Autodesk Fusion 360 part; units mm, degrees
(part 2 of 2)
sketch "草图2" plane through (0, 0, 0) normal (0, 0, 1) x (1, 0, 0)
  circle A0 centre (-78, 71) radius 2.1
  circle A1 centre (0, 135) radius 5
  circle A2 centre (-78, 101) radius 2.1
  circle A3 centre (6, 76.5) radius 1.5
  circle A4 centre (53, 101) radius 2.1
  arc A5 (8, 81) -> (8, 91) centre (8, 86) ccw
  line L0 (8, 81) -> (-8, 81)
  arc A6 (-8, 91) -> (-8, 81) centre (-8, 86) ccw
  line L1 (-8, 91) -> (8, 91)
  arc A7 (-116.45, 141.5) -> (-119.55, 141.5) centre (-118, 141.5) ccw
  line L2 (-116.45, 141.5) -> (-116.45, 131.5)
  arc A8 (-119.55, 131.5) -> (-116.45, 131.5) centre (-118, 131.5) ccw
  line L3 (-119.55, 131.5) -> (-119.55, 141.5)
  arc A9 (92, 50) -> (92, 53) centre (92, 51.5) ccw
  line L4 (92, 50) -> (87, 50)
  arc A10 (87, 53) -> (87, 50) centre (87, 51.5) ccw
  line L5 (87, 53) -> (92, 53)
  circle A11 centre (112.5, 146) radius 1.6
  arc A12 (75, 147.55) -> (75, 144.45) centre (75, 146) ccw
  line L6 (75, 147.55) -> (105, 147.55)
  arc A13 (105, 144.45) -> (105, 147.55) centre (105, 146) ccw
  line L7 (105, 144.45) -> (75, 144.45)
  circle A14 centre (78, 101) radius 2.1
  circle A15 centre (112, 140) radius 2.1
  circle A16 centre (22.5, 146) radius 1.6
  arc A17 (-15, 147.55) -> (-15, 144.45) centre (-15, 146) ccw
  line L8 (-15, 147.55) -> (15, 147.55)
  arc A18 (15, 144.45) -> (15, 147.55) centre (15, 146) ccw
  line L9 (15, 144.45) -> (-15, 144.45)
  arc A19 (30, 147.55) -> (30, 144.45) centre (30, 146) ccw
  line L10 (30, 147.55) -> (60, 147.55)
  arc A20 (60, 144.45) -> (60, 147.55) centre (60, 146) ccw
  line L11 (60, 144.45) -> (30, 144.45)
  arc A21 (-75, 144.45) -> (-75, 147.55) centre (-75, 146) ccw
  line L12 (-75, 144.45) -> (-105, 144.45)
  arc A22 (-105, 147.55) -> (-105, 144.45) centre (-105, 146) ccw
  line L13 (-105, 147.55) -> (-75, 147.55)
  circle A23 centre (-112.5, 146) radius 1.6
  circle A24 centre (-67.5, 146) radius 1.6
  circle A25 centre (-6, 76.5) radius 1.5
  circle A26 centre (-53, 71) radius 2.1
  circle A27 centre (35.5, 52.5) radius 1.5
  circle A28 centre (-45.5, 52.5) radius 1.5
  circle A29 centre (16, 54) radius 2.9
  circle A30 centre (67.5, 146) radius 1.6
  arc A31 (-60, 147.55) -> (-60, 144.45) centre (-60, 146) ccw
  line L14 (-60, 147.55) -> (-30, 147.55)
  arc A32 (-30, 144.45) -> (-30, 147.55) centre (-30, 146) ccw
  line L15 (-30, 144.45) -> (-60, 144.45)
  circle A33 centre (-16, 54) radius 2.9
  circle A34 centre (53, 71) radius 2.1
  circle A35 centre (45.5, 52.5) radius 1.5
  circle A36 centre (-35.5, 52.5) radius 1.5
  circle A37 centre (-40.5, 61) radius 5
  circle A38 centre (-53, 101) radius 2.1
  circle A39 centre (-14.0007, 100.9993) radius 1.3
  circle A40 centre (-22.5, 146) radius 1.6
  circle A41 centre (40.5, 61) radius 5
  circle A42 centre (78, 71) radius 2.1
  arc A43 (-87, 50) -> (-87, 53) centre (-87, 51.5) ccw
  line L16 (-87, 50) -> (-92, 50)
  arc A44 (-92, 53) -> (-92, 50) centre (-92, 51.5) ccw
  line L17 (-92, 53) -> (-87, 53)
  arc A45 (119.55, 141.5) -> (116.45, 141.5) centre (118, 141.5) ccw
  line L18 (119.55, 141.5) -> (119.55, 131.5)
  arc A46 (116.45, 131.5) -> (119.55, 131.5) centre (118, 131.5) ccw
  line L19 (116.45, 131.5) -> (116.45, 141.5)
  circle A47 centre (14.0007, 129.0007) radius 1.3
  circle A48 centre (-86, 58.5) radius 2.1
  circle A49 centre (86, 58.5) radius 2.1
  circle A50 centre (-86, 113.5) radius 2.1
  circle A51 centre (-91, 86) radius 2.1
  circle A52 centre (-40, 140) radius 2.1
  circle A53 centre (91, 86) radius 2.1
  circle A54 centre (86, 113.5) radius 2.1
  circle A55 centre (40, 140) radius 2.1
  circle A56 centre (14.0007, 100.9993) radius 1.3
  circle A57 centre (-14.0007, 129.0007) radius 1.3
  circle A58 centre (20.8597, 94.1403) radius 1.6
  circle A59 centre (-20.8597, 94.1403) radius 1.6
  circle A60 centre (-20.8597, 135.8597) radius 1.6
  circle A61 centre (20.8597, 135.8597) radius 1.6
  circle A62 centre (-112, 140) radius 2.1
  line L20 (-96, 123.5) -> (-96, 51.5)
  arc A63 (-96, 51.5) -> (-93, 48.5) centre (-93, 51.5) ccw
  line L21 (-93, 48.5) -> (93, 48.5)
  arc A64 (93, 48.5) -> (96, 51.5) centre (93, 51.5) ccw
  line L22 (96, 51.5) -> (96, 123.5)
  arc A65 (99, 126.5) -> (96, 123.5) centre (99, 123.5) ccw
  line L23 (99, 126.5) -> (117, 126.5)
  arc A66 (117, 126.5) -> (122, 131.5) centre (117, 131.5) ccw
  line L24 (122, 131.5) -> (122, 140)
  arc A67 (122, 140) -> (112, 150) centre (112, 140) ccw
  line L25 (112, 150) -> (-112, 150)
  arc A68 (-112, 150) -> (-122, 140) centre (-112, 140) ccw
  line L26 (-122, 140) -> (-122, 131.5)
  arc A69 (-122, 131.5) -> (-117, 126.5) centre (-117, 131.5) ccw
  line L27 (-117, 126.5) -> (-99, 126.5)
  arc A70 (-96, 123.5) -> (-99, 126.5) centre (-99, 123.5) ccw
  circle A71 centre (35.5, -52.5) radius 1.5
  circle A72 centre (-40.5, 33) radius 5
  circle A73 centre (45.5, -52.5) radius 1.5
  circle A74 centre (-35.5, -52.5) radius 1.5
  circle A75 centre (-45.5, -52.5) radius 1.5
  circle A76 centre (-39, -77) radius 1.6
  circle A77 centre (-39, -126) radius 1.6
  circle A78 centre (19, -77) radius 1.6
  circle A79 centre (19, -126) radius 1.6
  circle A80 centre (-19, -77) radius 1.6
  circle A81 centre (39, -77) radius 1.6
  circle A82 centre (39, -126) radius 1.6
  circle A83 centre (-19, -126) radius 1.6
  circle A84 centre (24.5, -62.5) radius 1.6
  circle A85 centre (24.5, -82.5) radius 1.6
  circle A86 centre (24.5, -120.5) radius 1.6
  circle A87 centre (24.5, -140.5) radius 1.6
  circle A88 centre (-24.5, -140.5) radius 1.6
  circle A89 centre (-24.5, -120.5) radius 1.6
  circle A90 centre (-24.5, -82.5) radius 1.6
  circle A91 centre (-24.5, -62.5) radius 1.6
  circle A92 centre (-5, -61.5) radius 1.5
  circle A93 centre (5, -61.5) radius 1.5
  circle A94 centre (-5, -35) radius 1.5
  circle A95 centre (5, -35) radius 1.5
  circle A96 centre (5, 35) radius 1.5
  circle A97 centre (-5, 35) radius 1.5
  circle A98 centre (35, 5) radius 1.5
  circle A99 centre (35, -5) radius 1.5
  circle A100 centre (-35, 5) radius 1.5
  circle A101 centre (-35, -5) radius 1.5
  circle A102 centre (-112.5, -146) radius 1.6
  arc A103 (-75, -147.55) -> (-75, -144.45) centre (-75, -146) ccw
  line L28 (-75, -147.55) -> (-105, -147.55)
  arc A104 (-105, -144.45) -> (-105, -147.55) centre (-105, -146) ccw
  line L29 (-105, -144.45) -> (-75, -144.45)
  arc A105 (-30, -147.55) -> (-30, -144.45) centre (-30, -146) ccw
  line L30 (-30, -147.55) -> (-60, -147.55)
  arc A106 (-60, -144.45) -> (-60, -147.55) centre (-60, -146) ccw
  line L31 (-60, -144.45) -> (-30, -144.45)
  circle A107 centre (-67.5, -146) radius 1.6
  arc A108 (-15, -144.45) -> (-15, -147.55) centre (-15, -146) ccw
  line L32 (-15, -144.45) -> (15, -144.45)
  arc A109 (15, -147.55) -> (15, -144.45) centre (15, -146) ccw
  line L33 (15, -147.55) -> (-15, -147.55)
  circle A110 centre (-22.5, -146) radius 1.6
  arc A111 (30, -144.45) -> (30, -147.55) centre (30, -146) ccw
  line L34 (30, -144.45) -> (60, -144.45)
  arc A112 (60, -147.55) -> (60, -144.45) centre (60, -146) ccw
  line L35 (60, -147.55) -> (30, -147.55)
  arc A113 (116.45, -141.5) -> (119.55, -141.5) centre (118, -141.5) ccw
  line L36 (116.45, -141.5) -> (116.45, -131.5)
  arc A114 (119.55, -131.5) -> (116.45, -131.5) centre (118, -131.5) ccw
  line L37 (119.55, -131.5) -> (119.55, -141.5)
  circle A115 centre (22.5, -146) radius 1.6
  arc A116 (75, -144.45) -> (75, -147.55) centre (75, -146) ccw
  line L38 (75, -144.45) -> (105, -144.45)
  arc A117 (105, -147.55) -> (105, -144.45) centre (105, -146) ccw
  line L39 (105, -147.55) -> (75, -147.55)
  circle A118 centre (-30.5, 30.5) radius 2.1
  circle A119 centre (67.5, -146) radius 1.6
  circle A120 centre (-112, -35.5) radius 2.1
  circle A121 centre (112.5, -146) radius 1.6
  arc A122 (-116.45, -131.5) -> (-119.55, -131.5) centre (-118, -131.5) ccw
  line L40 (-116.45, -131.5) -> (-116.45, -141.5)
  arc A123 (-119.55, -141.5) -> (-116.45, -141.5) centre (-118, -141.5) ccw
  line L41 (-119.55, -141.5) -> (-119.55, -131.5)
  circle A124 centre (-86, -113.5) radius 2.1
  line L42 (-102, 15) -> (-102, -15)
  arc A125 (-106, -15) -> (-102, -15) centre (-104, -15) ccw
  line L43 (-106, -15) -> (-106, 15)
  arc A126 (-102, 15) -> (-106, 15) centre (-104, 15) ccw
  circle A127 centre (-30.5, -30.5) radius 2.1
  circle A128 centre (-112, 35.5) radius 2.1
  arc A129 (-58, 15) -> (-62, 15) centre (-60, 15) ccw
  line L44 (-58, 15) -> (-58, -15)
  arc A130 (-62, -15) -> (-58, -15) centre (-60, -15) ccw
  line L45 (-62, -15) -> (-62, 15)
  circle A131 centre (91, -86) radius 2.1
  arc A132 (106, 15) -> (102, 15) centre (104, 15) ccw
  line L46 (106, 15) -> (106, -15)
  arc A133 (102, -15) -> (106, -15) centre (104, -15) ccw
  line L47 (102, -15) -> (102, 15)
  circle A134 centre (30.5, 30.5) radius 2.1
  circle A135 centre (-40, -140) radius 2.1
  circle A136 centre (30.5, -30.5) radius 2.1
  circle A137 centre (112, 35.5) radius 2.1
  circle A138 centre (86, -113.5) radius 2.1
  circle A139 centre (40, -140) radius 2.1
  arc A140 (62, 15) -> (58, 15) centre (60, 15) ccw
  line L48 (62, 15) -> (62, -15)
  arc A141 (58, -15) -> (62, -15) centre (60, -15) ccw
  line L49 (58, -15) -> (58, 15)
  circle A142 centre (112, -35.5) radius 2.1
  circle A143 centre (-91, -86) radius 2.1
  circle A144 centre (86, -58.5) radius 2.1
  circle A145 centre (-86, -58.5) radius 2.1
  circle A146 centre (-45.5, 41.5) radius 1.5
  circle A147 centre (-35.5, 41.5) radius 1.5
  circle A148 centre (-53, -101) radius 2.1
  arc A149 (-8, -81) -> (-8, -91) centre (-8, -86) ccw
  line L50 (-8, -81) -> (8, -81)
  arc A150 (8, -91) -> (8, -81) centre (8, -86) ccw
  line L51 (8, -91) -> (-8, -91)
  circle A151 centre (-118, -40) radius 1.6
  circle A152 centre (78, -101) radius 2.1
  circle A153 centre (22.5, 22.5) radius 1.55
  circle A154 centre (-118, 40) radius 1.6
  circle A155 centre (-15.25, 15.25) radius 1.55
  circle A156 centre (-22.5, -22.5) radius 1.55
  arc A157 (119.55, 32.5) -> (116.45, 32.5) centre (118, 32.5) ccw
  line L52 (119.55, 32.5) -> (119.55, 7.5)
  arc A158 (116.45, 7.5) -> (119.55, 7.5) centre (118, 7.5) ccw
  line L53 (116.45, 7.5) -> (116.45, 32.5)
  circle A159 centre (118, 40) radius 1.6
  circle A160 centre (118, 0) radius 1.6
  circle A161 centre (53, -101) radius 2.1
  circle A162 centre (15.25, -15.25) radius 1.55
  arc A163 (92, 41) -> (92, 44) centre (92, 42.5) ccw
  line L54 (92, 41) -> (87, 41)
  arc A164 (87, 44) -> (87, 41) centre (87, 42.5) ccw
  line L55 (87, 44) -> (92, 44)
  arc A165 (-87, 41) -> (-87, 44) centre (-87, 42.5) ccw
  line L56 (-87, 41) -> (-92, 41)
  arc A166 (-92, 44) -> (-92, 41) centre (-92, 42.5) ccw
  line L57 (-92, 44) -> (-87, 44)
  circle A167 centre (-78, -101) radius 2.1
  circle A168 centre (35.5, 41.5) radius 1.5
  circle A169 centre (-20.5, 39.5) radius 2.75
  circle A170 centre (20.5, 39.5) radius 2.75
  circle A171 centre (45.5, 41.5) radius 1.5
  circle A172 centre (-112, -140) radius 2.1
  circle A173 centre (-15.25, -15.25) radius 1.55
  circle A174 centre (22.5, -22.5) radius 1.55
  circle A175 centre (-118, 0) radius 1.6
  arc A176 (-116.45, -7.5) -> (-119.55, -7.5) centre (-118, -7.5) ccw
  line L58 (-116.45, -7.5) -> (-116.45, -32.5)
  arc A177 (-119.55, -32.5) -> (-116.45, -32.5) centre (-118, -32.5) ccw
  line L59 (-119.55, -32.5) -> (-119.55, -7.5)
  circle A178 centre (-53, -71) radius 2.1
  circle A179 centre (112, -140) radius 2.1
  arc A180 (-119.55, 7.5) -> (-116.45, 7.5) centre (-118, 7.5) ccw
  line L60 (-119.55, 7.5) -> (-119.55, 32.5)
  arc A181 (-116.45, 32.5) -> (-119.55, 32.5) centre (-118, 32.5) ccw
  line L61 (-116.45, 32.5) -> (-116.45, 7.5)
  circle A182 centre (0, 0) radius 1.6
  arc A183 (116.45, -32.5) -> (119.55, -32.5) centre (118, -32.5) ccw
  line L62 (116.45, -32.5) -> (116.45, -7.5)
  arc A184 (119.55, -7.5) -> (116.45, -7.5) centre (118, -7.5) ccw
  line L63 (119.55, -7.5) -> (119.55, -32.5)
  circle A185 centre (53, -71) radius 2.1
  circle A186 centre (40.5, 33) radius 5
  circle A187 centre (-22.5, 22.5) radius 1.55
  circle A188 centre (-40.5, -61) radius 5
  circle A189 centre (-78, -71) radius 2.1
  circle A190 centre (40.5, -61) radius 5
  circle A191 centre (118, -40) radius 1.6
  circle A192 centre (15.25, 15.25) radius 1.55
  circle A193 centre (78, -71) radius 2.1
  arc A194 (-117, 45.5) -> (-122, 40.5) centre (-117, 40.5) ccw
  line L64 (-122, 40.5) -> (-122, -40.5)
  arc A195 (-122, -40.5) -> (-117, -45.5) centre (-117, -40.5) ccw
  line L65 (-117, -45.5) -> (-99, -45.5)
  arc A196 (-96, -48.5) -> (-99, -45.5) centre (-99, -48.5) ccw
  line L66 (-96, -48.5) -> (-96, -123.5)
  arc A197 (-99, -126.5) -> (-96, -123.5) centre (-99, -123.5) ccw
  line L67 (-99, -126.5) -> (-117, -126.5)
  arc A198 (-117, -126.5) -> (-122, -131.5) centre (-117, -131.5) ccw
  line L68 (-122, -131.5) -> (-122, -140)
  arc A199 (-122, -140) -> (-112, -150) centre (-112, -140) ccw
  line L69 (-112, -150) -> (112, -150)
  arc A200 (112, -150) -> (122, -140) centre (112, -140) ccw
  line L70 (122, -140) -> (122, -131.5)
  arc A201 (122, -131.5) -> (117, -126.5) centre (117, -131.5) ccw
  line L71 (117, -126.5) -> (99, -126.5)
  arc A202 (96, -123.5) -> (99, -126.5) centre (99, -123.5) ccw
  line L72 (96, -123.5) -> (96, -48.5)
  arc A203 (99, -45.5) -> (96, -48.5) centre (99, -48.5) ccw
  line L73 (99, -45.5) -> (117, -45.5)
  arc A204 (117, -45.5) -> (122, -40.5) centre (117, -40.5) ccw
  line L74 (122, -40.5) -> (122, 40.5)
  arc A205 (122, 40.5) -> (117, 45.5) centre (117, 40.5) ccw
  line L75 (117, 45.5) -> (-117, 45.5)
equation "d26 = ( 32 / 2 ) * 1 mm"
equation "d51 = ( 41 / 2 ) * 1 mm"
equation "d57 = 5.5 mm + 0.3 mm"
equation "d59 = ( 32 / 2 ) * 1 mm"
equation "d63 = ( 30.5 / 2 ) * 1 mm"
equation "d64 = ( 45 / 2 ) * 1 mm"
equation "d116 = ( 12 / 2 ) * 1 mm"
